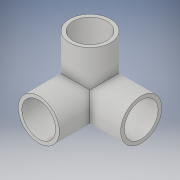
# Autodesk Inventor part: 3-way 90 1 Inch
Saved by Autodesk Inventor 2018 (Build 220112000, 112)
## iProperties
Created: 2018-01-18
Part Number: 3-way 90 1 Inch
Material: Generic
Document SubType Name: Modeling
Designer: owner
Density: 1 g/cm^3
Appearance: Default
Author: owner
Autodesk Inventor part; units mm, degrees
ref_plane "YZ Plane" through (0, 0, 0) normal (1, 0, 0) x (0, 1, 0)
sketch "Sketch18" plane through (0, 0, 0) normal (0, 0, 1) x (1, 0, 0)
  circle A0 centre (0, 0) radius 20.3835
  dimension "d50" = 40.767
  constraints: 1 centre point, 1 coincident
  measures "d50" diameter of A0
extrude "Extrusion10" add sketch "Sketch18" against normal blind 50.8
sketch "Sketch24" plane through (0, 0, 0) normal (0, 0, 1) x (1, 0, 0)
  line L0 (0, 0) -> (20.3835, 0)
  circle A0 centre (0, 0) radius 20.3835 projected
  line L1 (0, 0) -> (0, 20.3835)
  constraints: 4 end point, 2 point on circle, 1 horizontal, 1 perpendicular
ref_plane "Work Plane16" through (0, 0, 0) normal (1, 0, 0) x (0, 1, 0)
ref_plane "Work Plane17" through (0, 0, 0) normal (0, -1, 0) x (1, 0, 0)
sketch "Sketch25" plane through (0, 0, 0) normal (1, 0, 0) x (0, 1, 0)
  line L0 (-20.3835, -50.8) -> (20.3835, -50.8) projected
  circle A0 centre (0, -50.8) radius 20.3835
  point P0 (0, 0)
  dimension "d67" = 40.767
  constraints: 1 centre point, 1 midpoint
  measures "d67" diameter of A0
sketch "Sketch26" plane through (0, 0, 0) normal (0, -1, 0) x (1, 0, 0)
  line L0 (-20.3835, -50.8) -> (20.3835, -50.8) projected
  circle A0 centre (0, -50.8) radius 20.3835
  point P0 (0, 0)
  constraints: 1 horizontal alignment, 1 midpoint, 2 other
extrude "Extrusion14" add sketch "Sketch26" against normal blind 50.8
extrude "Extrusion15" add sketch "Sketch25" along normal blind 50.8
sketch "Sketch27" plane through (0, 0, 0) normal (-1, 0, 0) x (0, 0, 1)
  line L0 (-50.8, 0) -> (-50.8, -20.3835) projected
  line L1 (-50.8, 0) -> (-50.8, -20.3835)
  circle A0 centre (-50.8, 0) radius 20.3835 projected
  line L2 (-50.8, 0) -> (-71.1835, 0) projected
  line L3 (-50.8, 0) -> (-71.1835, 0)
  arc A1 (-71.1835, 0) -> (-50.8, -20.3835) centre (-50.8, 0) ccw
  point P0 (0, 0)
  constraints: 4 end point, 3 point on circle, 1 centre point, 1 coincident, 1 collinear, 1 vertical
revolve "Revolution12" add sketch "Sketch27" angle 90 about axis through (0, 0, -50.8) along (0, 1, 0) picked at (-52.3119, -13.4186) contours L0 A0 L2
sketch "Sketch28" plane through (0, 0, 0) normal (0, 0, 1) x (1, 0, 0)
  line L0 (20.3835, 20.3835) -> (0, 0) projected
  circle A0 centre (0, 0) radius 12.7
  line L1 (0, 0) -> (0, -20.3835) projected
  circle A1 centre (0, 0) radius 16.7767
  point P0 (14.4133, 14.4133)
  dimension "d73" = 25.4
  dimension "d74" = 33.5534
  constraints: 2 centre point, 2 coincident
  measures "d73" diameter of A0
  measures "d74" diameter of A1
sketch "Sketch29" plane through (0, 50.8, -50.8) normal (0, 1, 0) x (1, 0, 0)
  line L0 (0, 20.3835) -> (0, 0) projected
  circle A0 centre (0, 0) radius 12.7
  line L1 (0, 0) -> (-20.3835, 0) projected
  circle A1 centre (0, 0) radius 16.7767
  point P0 (0, -50.8)
  dimension "d75" = 25.4
  dimension "d76" = 33.5534
  constraints: 2 centre point, 1 coincident
  measures "d75" diameter of A0
  measures "d76" diameter of A1
sketch "Sketch30" plane through (50.8, 0, -50.8) normal (1, 0, 0) x (0, 0, -1)
  circle A0 centre (0, 0) radius 20.3835 projected
  circle A1 centre (0, 0) radius 12.7
  line L0 (-20.3835, 20.3835) -> (0, 0) projected
  circle A2 centre (0, 0) radius 16.7767
  point P0 (-50.8, 0)
  point P1 (-14.4133, 14.4133)
  dimension "d77" = 25.4
  dimension "d78" = 33.5534
  constraints: 2 centre point, 2 coincident, 1 other
  measures "d77" diameter of A1
  measures "d78" diameter of A2
extrude "Extrusion16" cut sketch "Sketch30" against normal blind 50.8 contours A1
extrude "Extrusion17" cut sketch "Sketch28" against normal blind 50.8 contours A0 L1 L0 | L0 L1 A0
extrude "Extrusion18" cut sketch "Sketch29" against normal blind 50.8 contours A0 L1 L0 | L0 L1 A0
extrude "Extrusion19" cut sketch "Sketch30" against normal blind 31.75 contours A2
extrude "Extrusion20" cut sketch "Sketch28" against normal blind 31.75 contours A1 L1 A0 L0 | L0 A0 L1 A1
extrude "Extrusion21" cut sketch "Sketch29" against normal blind 31.75 contours A1 L1 A0 L0 | L0 A0 L1 A1
sketch "Sketch31" plane through (0, 0, -50.8) normal (1, 0, 0) x (0, 0, -1)
  line L0 (12.7, 0) -> (0, 0) projected
  line L1 (0, 0) -> (0, -12.7) projected
  arc A0 (0, -12.7) -> (12.7, 0) centre (0, 0) ccw projected
  point P0 (-50.8, 0)
revolve "Revolution13" cut sketch "Sketch31" angle 90 about axis through (0, 0, -50.8) along (0, 1, 0)
body "Solid3"
